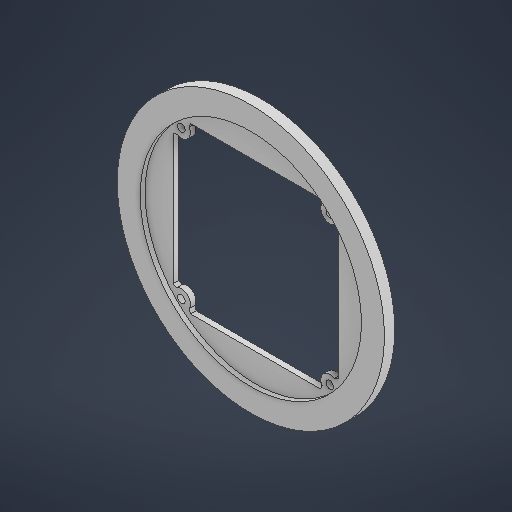
# Autodesk Inventor part: moteus_x1_mount
Saved by Autodesk Inventor 2026.1 (Build 301233000, 233)
## iProperties
Created: 2026-04-28
Part Number: moteus_x1_mount
Material: Generic
Document SubType Name: Modeling
Designer: aaron
Density: 1 g/cm^3
Appearance: Default
Author: aaron
Autodesk Inventor part; units mm, degrees
ref_plane "YZ Plane" through (0, 0, 0) normal (1, 0, 0) x (0, 1, 0)
ref_plane "XZ Plane" through (0, 0, 0) normal (0, 1, 0) x (-1, 0, 0)
ref_plane "XY Plane" through (0, 0, 0) normal (0, 0, 1) x (1, 0, 0)
sketch "Sketch1" plane through (0, 0, 0) normal (0, 0, 1) x (1, 0, 0)
  line L0 (-25, 25) -> (25, 25)
  line L1 (25, 25) -> (25, -25)
  line L2 (25, -25) -> (-25, -25)
  line L3 (-25, -25) -> (-25, 25)
  circle A0 centre (-25, 25) radius 1.25
  circle A1 centre (-25, 25) radius 3
  circle A2 centre (-25, -25) radius 3
  circle A3 centre (-25, -25) radius 1.25
  circle A4 centre (25, -25) radius 3
  circle A5 centre (25, -25) radius 1.25
  circle A6 centre (25, 25) radius 3
  circle A7 centre (25, 25) radius 1.25
  circle A8 centre (0, 0) radius 45
  line L4 (27.8, 27.8) -> (-27.8, 27.8)
  line L5 (-27.8, 27.8) -> (-27.8, -27.8)
  line L6 (-27.8, -27.8) -> (27.8, -27.8)
  line L7 (27.8, -27.8) -> (27.8, 27.8)
  point P0 (-22, 25)
  point P1 (22, 25)
  point P2 (25, 22)
  point P3 (25, -22)
  point P4 (22, -25)
  point P5 (-22, -25)
  point P6 (-25, -22)
  point P7 (-25, 22)
  point P8 (-23.923, 27.8)
  point P9 (23.923, 27.8)
  point P10 (27.8, 23.923)
  point P11 (27.8, -23.923)
  point P12 (23.923, -27.8)
  point P13 (-23.923, -27.8)
  point P14 (-27.8, -23.923)
  point P15 (-27.8, 23.923)
  dimension "d0" = 50
  dimension "d1" = 25
  dimension "d2" = 50
  dimension "d3" = 25
  dimension "d4" = 2.5
  dimension "d5" = 6
  dimension "d8" = 360
  dimension "d12" = 90
  dimension "d14" = 2.8
  constraints: 16 end point, 9 centre point, 6 coincident, 4 parallel, 2 perpendicular, 1 horizontal, 20 other
  measures "d0" distance of L0.start L0.end
  measures "d1" distance from line of L0 point (0, 0)
  measures "d2" distance of L2.end L0.start
  measures "d3" distance from line of L3 point (0, 0)
  measures "d4" diameter of A0
  measures "d5" diameter of A1
  measures "d12" diameter of A8
  measures "d14" distance between parallel lines of L4 L0
extrude "Extrusion1" add sketch "Sketch1" along normal blind 3.5 contours A0 L3 A1 L5 L4 L0 | L0 A1 L3 A0 | A6 L4 L7 L1 A7 L0 | L0 A7 L1 A6 | L4 A1 | A2 L2 A3 L3 | L3 A3 L2 A2 L6 L5 | A1 L5 | A6 L4 | A1 L5 L4 | L5 A2 | L4 L7 A6 | A4 L7 L6 L2 A5 L1 | L1 A5 L2 A4 | L7 A6 | A2 L6 | A2 L6 L5 | A4 L7 | L6 A4 | L7 L6 A4 | A8
chamfer "Chamfer1" distance 2 angle 45 8 edges at (-23.923, -27.8, 1.75) (-27.8, -23.923, 1.75) (23.923, -27.8, 1.75) (27.8, -23.923, 1.75) (23.923, 27.8, 1.75) (27.8, 23.923, 1.75) (-23.923, 27.8, 1.75) (-27.8, 23.923, 1.75)
sketch "Sketch2" plane through (0, 0, 3.5) normal (0, 0, 1) x (1, 0, 0)
  circle A0 centre (0, 0) radius 37.25
  dimension "d18" = 74.5
  constraints: 1 centre point, 1 coincident
  measures "d18" diameter of A0
extrude "Extrusion2" cut sketch "Sketch2" against normal blind 1.6
sketch "Sketch3" plane through (0, 0, 0) normal (0, 0, -1) x (-1, 0, 0)
  circle A0 centre (-17.9346, -27.7011) radius 1.65 projected
  circle A1 centre (15.0226, -29.3824) radius 1.65 projected
  circle A2 centre (15.0226, -29.3824) radius 1.65
  circle A3 centre (32.9571, -1.6813) radius 1.65
  circle A4 centre (17.9346, 27.7011) radius 1.65
  circle A5 centre (-15.0226, 29.3824) radius 1.65
  circle A6 centre (-32.9571, 1.6813) radius 1.65
  circle A7 centre (-17.9346, -27.7011) radius 1.65
  point P0 (0, 0)
  dimension "d23" = 360
  constraints: 6 centre point, 1 coincident, 1 concentric, 13 other
equation "\"d1\" = 0.5 * d0"
equation "\"d2\" = d0"
equation "\"d3\" = d1"
body "Solid1"
